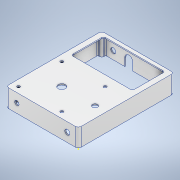
# Autodesk Inventor part: Ventilator Base 01
Saved by Autodesk Inventor 2021 (Build 250183000, 183)
## iProperties
Created: 2020-04-14
Part Number: Ventilator Base 01
Material: PAEK Plastic
Document SubType Name: Modeling
Designer: James
Density: 1.32 g/cm^3
Appearance: Aluminum - Flat
Author: James
Autodesk Inventor part; units mm, degrees
ref_plane "YZ Plane" through (0, 0, 0) normal (1, 0, 0) x (0, 1, 0)
ref_plane "XZ Plane" through (0, 0, 0) normal (0, 1, 0) x (-1, 0, 0)
ref_plane "XY Plane" through (0, 0, 0) normal (0, 0, 1) x (1, 0, 0)
sketch "Sketch1" plane through (0, 0, 0) normal (0, 1, 0) x (-1, 0, 0)
  line L0 (0, 0) -> (200, 0)
  line L1 (200, 0) -> (200, -265)
  line L2 (200, -265) -> (0, -265)
  line L3 (0, -265) -> (0, 0)
  dimension "d0" = 265
  dimension "d1" = 200
  constraints: 8 end point, 2 horizontal, 2 parallel, 1 perpendicular
  measures "d0" distance of L0.end L1.end
  measures "d1" distance of L1.end L2.end
extrude "Extrusion1" add sketch "Sketch1" along normal blind 50
sketch "Sketch2" plane through (0, 50, 0) normal (0, 1, 0) x (1, 0, 0)
  line L0 (-62, 136.5) -> (-182, 136.5)
  line L1 (-182, 136.5) -> (-182, 16.5)
  line L2 (-182, 16.5) -> (-62, 16.5)
  line L3 (-62, 16.5) -> (-62, 136.5)
  line L4 (-200, 0) -> (0, 0) projected
  line L5 (-200, 265) -> (-200, 0) projected
  circle A0 centre (-62, 16.5) radius 4
  circle A1 centre (-182, 16.5) radius 4
  circle A2 centre (-62, 136.5) radius 4
  circle A3 centre (-182, 136.5) radius 4
  line L6 (-62, 16.5) -> (-60.5, 16.5)
  dimension "d13" = 120
  dimension "d14" = 120
  dimension "d17" = 8
  dimension "d18" = 8
  dimension "d19" = 8
  dimension "d20" = 8
  dimension "d74" = 1.5
  constraints: 10 end point, 4 centre point, 4 coincident, 2 horizontal, 2 parallel, 1 perpendicular
  measures "d13" distance of L1.end L2.end
  measures "d14" distance of L2.end L0.start
  measures "d17" diameter of A0
  measures "d18" diameter of A1
  measures "d19" diameter of A2
  measures "d20" diameter of A3
  measures "d74" distance of L6.start L6.end
fillet "Fillet1" radius 8 4 edges at (-200, 25, -265) (0, 25, -265) (-200, 25, 0) (0, 25, 0)
sketch "Sketch3" plane through (0, 0, 0) normal (0, -1, 0) x (1, 0, 0)
  point P0 (0, 0)
shell "Shell3" thickness 3 removed faces 1 at (-66.6667, 0, -91)
fillet "Fillet2" radius 5 8 edges at (-195.5355, 47, -4.4645) (-100, 47, -3) (-4.4645, 47, -4.4645) (-3, 47, -132.5) (-4.4645, 47, -260.5355) (-100, 47, -262) (-195.5355, 47, -260.5355) (-197, 47, -132.5)
extrude "Extrusion2" cut sketch "Sketch2" against normal blind 5 contours A3 L1 L0 | L0 L1 A3 | A2 L3 L0 | L0 L3 A2 | A1 L2 L1 | L1 L2 A1 | A0 L2 L3 | L3 L2 A0
sketch "Sketch6" plane through (0, 50, 0) normal (0, 1, 0) x (1, 0, 0)
  circle A0 centre (-122, 76.5) radius 10
  line L0 (-200, 257) -> (-200, 8) projected
  line L1 (-192, 3) -> (-8, 3) projected
  line L2 (-192, 0) -> (-217.2628, 0)
  line L3 (-192, 0) -> (-8, 0) projected
  point P0 (0, 0)
  dimension "d33" = 20
  constraints: 2 end point, 1 centre point, 1 horizontal
  measures "d33" diameter of A0
extrude "Extrusion5" cut sketch "Sketch6" against normal blind 5
sketch "Sketch8" plane through (-8, 0, -265) normal (0, 0, -1) x (-1, 0, 0)
  line L0 (184, 0) -> (0, 0) projected
  arc A0 (125, 22) -> (103, 22) centre (114, 22) ccw
  line L1 (104, 50) -> (104, 47) projected
  line L2 (104, 48.5) -> (124, 48.5)
  line L3 (124, 50) -> (124, 47) projected
  circle A1 centre (157, 22) radius 7
  line L4 (192, 0) -> (192, 50) projected
  line L5 (192, 0) -> (184, 0) projected
  line L6 (103, 22) -> (103, 0)
  line L7 (125, 22) -> (125, 0)
  line L8 (0, 0) -> (184, 0) projected
  line L9 (103, 0) -> (125, 0)
  point P0 (-8, 0)
  dimension "d45" = 22
  dimension "d46" = 22
  dimension "d50" = 14
  dimension "d51" = 35
  dimension "d71" = 78
  dimension "d77" = 22
  constraints: 8 end point, 2 centre point, 2 midpoint, 2 perpendicular, 2 point on circle, 2 point on line, 1 collinear
  measures "d45" diameter of A0
  measures "d46" distance from line of L0 A0.centre
  measures "d50" diameter of A1
  measures "d51" distance from line of L4 A1.centre
  measures "d71" distance from line of L4 A0.centre
  measures "d77" distance from line of L5 A1.centre
extrude "Extrusion6" cut sketch "Sketch8" against normal blind 5
sketch "Sketch9" plane through (0, 50, 0) normal (0, 1, 0) x (1, 0, 0)
  circle A0 centre (-122, 76.5) radius 10 projected
  line L0 (-122, 76.5) -> (32.3388, 76.5)
  circle A1 centre (-30, 76.5) radius 7
  line L1 (0, 8) -> (0, 257) projected
  point P0 (0, 0)
  dimension "d52" = 14
  dimension "d53" = 30
  constraints: 2 end point, 1 centre point, 1 horizontal, 1 point on line
  measures "d52" diameter of A1
  measures "d53" distance from line of L1 A1.centre
extrude "Extrusion7" cut sketch "Sketch9" against normal blind 5 contours A1 L0 | L0 A1
sketch "Sketch10" plane through (-192, 0, 0) normal (0, 0, 1) x (1, 0, 0)
  circle A0 centre (162, 25) radius 7
  line L0 (0, 0) -> (184, 0) projected
  line L1 (155, 50) -> (155, 47) projected
  line L2 (169, 50) -> (169, 47) projected
  point P0 (192, 0)
  dimension "d56" = 14
  dimension "d57" = 25
  constraints: 1 centre point
  measures "d56" diameter of A0
  measures "d57" distance from line of A0.centre L0
extrude "Extrusion8" cut sketch "Sketch10" against normal blind 5
sketch "Sketch11" plane through (0, 50, 0) normal (0, 1, 0) x (1, 0, 0)
  line L0 (-185, 255) -> (-15, 255)
  line L1 (-15, 255) -> (-15, 165)
  line L2 (-15, 165) -> (-185, 165)
  line L3 (-185, 165) -> (-185, 255)
  line L4 (-200, 257) -> (-200, 8) projected
  line L5 (0, 8) -> (0, 257) projected
  line L6 (-8, 265) -> (-192, 265) projected
  point P0 (0, 0)
  dimension "d64" = 90
  dimension "d65" = 15
  dimension "d66" = 15
  dimension "d67" = 10
  constraints: 8 end point, 3 perpendicular, 1 horizontal
  measures "d64" distance of L0.end L1.end
  measures "d65" distance between parallel lines of L4 L3
  measures "d66" distance between parallel lines of L5 L1
  measures "d67" distance between parallel lines of L6 L0
extrude "Extrusion9" cut sketch "Sketch11" against normal blind 10
fillet "Fillet3" radius 6 4 edges at (-185, 48.5, -165) (-185, 48.5, -255) (-15, 48.5, -165) (-15, 48.5, -255)
sketch "Sketch12" plane through (0, 0, 0) normal (0, -1, 0) x (1, 0, 0)
  line L0 (-3, -8) -> (-3, -257) projected
  line L1 (-3, -257) -> (-3, -8) projected
  circle A0 centre (-8, -257) radius 2
  line L2 (-6, -255.5) -> (-6, -255.5)
  line L3 (-9.5, -259) -> (-9.5, -259)
  line L4 (-100, 0) -> (-100, 40.5993)
  line L5 (-197, -8) -> (-197, -257)
  line L6 (-197, -257) -> (-197, -8)
  line L7 (-197, -251.1271) -> (-197, -252.5)
  line L8 (-8, -259) -> (-8, -257)
  arc A1 (-8, -251) -> (-14, -257) centre (-8, -257) ccw
  line L9 (-8, -8) -> (-8, -257) projected
  line L10 (-8, -251) -> (-6, -251)
  line L11 (-8, -257) -> (-192, -257) projected
  line L12 (-14, -257) -> (-14, -259)
  line L13 (-192, -262) -> (-8, -262) projected
  arc A2 (-6, -251) -> (-3, -248) centre (-6, -248) ccw
  arc A3 (-17, -262) -> (-14, -259) centre (-17, -259) ccw
  line L14 (-3, -248) -> (-3, -262)
  line L15 (-3, -262) -> (-17, -262)
  line L16 (-100, -262) -> (-100, -286.7332)
  line L17 (-190.5, -259) -> (-190.5, -259)
  line L18 (-194, -255.5) -> (-194, -255.5)
  circle A4 centre (-192, -257) radius 2
  line L19 (-192, -259) -> (-192, -257)
  arc A5 (-186, -257) -> (-192, -251) centre (-192, -257) ccw
  line L20 (-192, -251) -> (-194, -251)
  line L21 (-186, -257) -> (-186, -259)
  arc A6 (-197, -248) -> (-194, -251) centre (-194, -248) ccw
  arc A7 (-186, -259) -> (-183, -262) centre (-183, -259) ccw
  line L22 (-197, -248) -> (-197, -262)
  line L23 (-197, -262) -> (-183, -262)
  line L24 (0, -8) -> (0, -257) projected
  line L25 (0, -132.5) -> (85.796, -132.5)
  line L26 (-194, -116.5) -> (31.6393, -116.5)
  arc A8 (-6, -150.5) -> (-3, -147.5) centre (-6, -147.5) ccw
  arc A9 (-3, -165.5) -> (-6, -162.5) centre (-6, -165.5) ccw
  line L27 (-6, -156.5) -> (-8, -156.5)
  circle A10 centre (-8, -156.5) radius 2
  arc A11 (-8, -150.5) -> (-8, -162.5) centre (-8, -156.5) ccw
  line L28 (-6, -162.5) -> (-8, -162.5)
  line L29 (-6, -150.5) -> (-8, -150.5)
  line L30 (-3, -165.5) -> (-3, -147.5)
  arc A12 (-197, -147.5) -> (-194, -150.5) centre (-194, -147.5) ccw
  arc A13 (-194, -162.5) -> (-197, -165.5) centre (-194, -165.5) ccw
  line L31 (-194, -156.5) -> (-192, -156.5)
  circle A14 centre (-192, -156.5) radius 2
  arc A15 (-192, -162.5) -> (-192, -150.5) centre (-192, -156.5) ccw
  line L32 (-194, -162.5) -> (-192, -162.5)
  line L33 (-194, -150.5) -> (-192, -150.5)
  line L34 (-197, -165.5) -> (-197, -147.5)
  line L35 (31.6393, -116.5) -> (31.6393, -151.5)
  line L36 (31.6393, -151.5) -> (31.6393, -156.5)
  line L37 (-219.3128, -38.8787) -> (-219.3128, -151.5)
  line L38 (-192, -156.5) -> (-219.3128, -156.5)
  arc A16 (-6, -29) -> (-3, -26) centre (-6, -26) ccw
  arc A17 (-3, -44) -> (-6, -41) centre (-6, -44) ccw
  line L39 (-6, -35) -> (-8, -35)
  circle A18 centre (-8, -35) radius 2
  arc A19 (-8, -29) -> (-8, -41) centre (-8, -35) ccw
  line L40 (-6, -41) -> (-8, -41)
  line L41 (-6, -29) -> (-8, -29)
  line L42 (-3, -44) -> (-3, -26)
  arc A20 (-197, -26) -> (-194, -29) centre (-194, -26) ccw
  line L43 (-194, -35) -> (-192, -35)
  line L44 (-194, -29) -> (-192, -29)
  circle A21 centre (-192, -35) radius 2
  arc A22 (-192, -41) -> (-192, -29) centre (-192, -35) ccw
  line L45 (-194, -41) -> (-192, -41)
  line L46 (-197, -44) -> (-197, -26)
  arc A23 (-194, -41) -> (-197, -44) centre (-194, -44) ccw
  line L47 (-219.3128, -38.8787) -> (-219.3128, -33.8787)
  line L48 (-192, 0) -> (-8, 0) projected
  line L49 (-133, -265) -> (-192, -265) projected
  line L50 (-8, 0) -> (16.1683, 0)
  point P0 (-4, -232)
  point P1 (-4, -212)
  point P2 (-3, -257)
  point P3 (-8, -265)
  point P4 (-5, -271.0975)
  point P5 (-192, -3)
  point P6 (-8, -3)
  point P7 (-196, -212)
  point P8 (-196, -232)
  point P9 (-3, -251)
  point P10 (-14, -262)
  point P11 (-200, -257)
  point P12 (-195, -271.0975)
  point P13 (-197, -251)
  point P14 (-186, -262)
  point P15 (-3, -165.5)
  point P16 (-3, -147.5)
  point P17 (-8, -262)
  point P18 (-3, -257)
  point P19 (-200, -132.5)
  point P20 (-197, -147.5)
  point P21 (-197, -165.5)
  point P22 (-3, -44)
  point P23 (-3, -26)
  point P24 (-197, -26)
  point P25 (-197, -44)
  dimension "d134" = 2
  dimension "d135" = 4
  dimension "d136" = 3
  dimension "d138" = 4
  dimension "d145" = 3
  dimension "d167" = 2
  dimension "d168" = 4
  dimension "d169" = 4
  dimension "d171" = 35
  dimension "d172" = 5
  dimension "d174" = 3
  dimension "d175" = 2
  dimension "d176" = 4
  dimension "d177" = 4
  dimension "d179" = 5
  dimension "d186" = 8
  dimension "d187" = 108.5
  dimension "d189" = 35
  dimension "d190" = 35
  constraints: 82 end point, 36 point on circle, 28 symmetric about line, 24 centre point, 8 vertical, 6 point on line, 5 horizontal, 4 coincident, 4 tangent, 3 equal radius, 2 midpoint, 2 perpendicular, 13 other
  measures "d134" distance of L8.start L8.end
  measures "d135" radial gap between concentric circles of A0 A1
  measures "d136" radius of A2
  measures "d138" diameter of A0
  measures "d145" radius of A8
  measures "d167" distance of L27.start L27.end
  measures "d168" diameter of A10
  measures "d169" radial gap between concentric circles of A10 A11
  measures "d171" distance of L26.end L35.end
  measures "d172" distance of L35.end L36.end
  measures "d174" radius of A16
  measures "d175" distance of L39.start L39.end
  measures "d176" diameter of A18
  measures "d177" radial gap between concentric circles of A18 A19
  measures "d179" distance of L37.start L47.end
  measures "d186" distance from line of L11.end L49
  measures "d187" distance from line of L31.end L49
  measures "d189" distance from line of L48 A21.centre
  measures "d190" distance from line of L48 A18.centre
sketch "Sketch14" plane through (-192, 0, 0) normal (0, 0, 1) x (1, 0, 0)
  circle A0 centre (162, 25) radius 7 projected
  line L0 (162, 25) -> (-43.7697, 25)
  circle A1 centre (22, 25) radius 6
  point P0 (192, 0)
  point P1 (192, 50)
  point P2 (-8, 50)
  dimension "d126" = 12
  constraints: 2 end point, 1 centre point, 1 horizontal
  measures "d126" diameter of A1
extrude "Extrusion14" cut sketch "Sketch14" against normal blind 30 contours A1 L0 | L0 A1
extrude "Extrusion15" add sketch "Sketch12" against normal up to surface (47 mm away) contours L0 A17 L40 L9 A18 L41 A16 | L9 A18 A19 | L0 A9 L28 L9 A10 L29 A8 | A18 L39 L9 | L9 A18 | L9 A10 A11 | L9 L39 A18 | L0 L14 L15 L13 A3 L12 L11 A0 L9 L10 A2 | A10 L27 L9 | L9 A10 | L27 A10 L9 | L9 A0 L11 A1 | L9 L11 A0 | A0 L8 L9 | L21 A7 L13 L23 L22 L5 A6 L20 A5 | L11 L8 A0 | A20 L44 A22 L45 A23 L5 | A12 L33 A15 L32 A13 L5 | A4 L19 L11 | L11 L19 A4 | A14 | A21
sketch "Sketch15" plane through (0, 0, 0) normal (0, -1, 0) x (1, 0, 0)
  arc A0 (-8, -251) -> (-14, -257) centre (-8, -257) ccw projected
  circle A1 centre (-8, -257) radius 1.65
  circle A2 centre (-192, -257) radius 1.65
  arc A3 (-8, -150.5) -> (-8, -162.5) centre (-8, -156.5) ccw projected
  circle A4 centre (-8, -156.5) radius 1.65
  arc A5 (-192, -162.5) -> (-192, -150.5) centre (-192, -156.5) ccw projected
  circle A6 centre (-192, -156.5) radius 1.65
  line L0 (-8, -29) -> (-6, -29) projected
  line L1 (-6, -41) -> (-8, -41) projected
  line L2 (-8, -41) -> (-8, -150.5) projected
  line L3 (-8, -29) -> (-8, -41)
  arc A7 (-8, -29) -> (-8, -41) centre (-8, -35) ccw projected
  line L4 (-14, -35) -> (-8, -35)
  circle A8 centre (-8, -35) radius 1.65
  circle A9 centre (-192, -35) radius 1.65
  point P0 (0, 0)
  point P1 (-8, -8)
  dimension "d159" = 3.3
  dimension "d160" = 3.3
  dimension "d181" = 3.3
  dimension "d182" = 3.3
  dimension "d191" = 3.3
  dimension "d192" = 3.3
  constraints: 6 centre point, 4 coincident, 4 end point, 1 horizontal, 1 point on circle, 1 vertical
  measures "d159" diameter of A1
  measures "d160" diameter of A2
  measures "d181" diameter of A4
  measures "d182" diameter of A6
  measures "d191" diameter of A8
  measures "d192" diameter of A9
extrude "Extrusion16" cut sketch "Sketch15" against normal blind 30 contours A1 | A2 | A4 | A6 | A8 L3 | L3 L4 A8 | L3 A8 L4 | A9
sketch "Sketch16" plane through (0, 0, 0) normal (0, -1, 0) x (1, 0, 0)
  point P0 (0, 0)
fillet "Fillet5" radius 2 31 edges at (-6.9785, 46.8945, -251) (-3.6353, 44.4391, -249.8461) (-14, 46.8945, -258.0215) (-15.154, 44.439, -261.3648) (-12.2426, 47, -252.7574) (-186, 46.8945, -258.0215) (-184.8442, 44.4364, -261.3662) (-193.0215, 46.8945, -251) (-196.3647, 44.4391, -249.8461) (-187.7574, 47, -252.7574) (-193.0215, 46.8945, -162.5) (-196.3647, 44.4391, -163.6539) (-193.0215, 46.8945, -150.5) (-196.3647, 44.4391, -149.3461) (-186, 47, -156.5) (-6.9785, 46.8945, -150.5) (-3.6338, 44.4364, -149.3442) (-6.9785, 46.8945, -162.5) (-3.6352, 44.439, -163.654) (-14, 47, -156.5) (-193.0215, 46.8945, -29) (-193.0215, 46.8945, -41) (-196.3647, 44.4391, -27.8461) (-196.3647, 44.4391, -42.1539) (-100, 47, -8) (-186, 47, -35) (-6.9785, 46.8945, -41) (-6.9785, 46.8945, -29) (-3.6352, 44.439, -42.154) (-3.6338, 44.4364, -27.8442) (-14, 47, -35)
fillet_without_effect "Fillet6"
body "Solid1"
